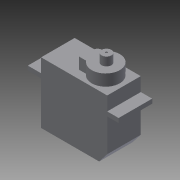
# Autodesk Inventor part: Part1
Saved by Autodesk Inventor 2015 (Build 190159000, 159)
## iProperties
Created: 2015-05-19
Part Number: Part1
Material: Generic
Document SubType Name: Modeling
Designer: Angelina
Density: 1 g/cm^3
Appearance: Default
Author: Angelina
Autodesk Inventor part; units mm, degrees
ref_plane "YZ Plane" through (0, 0, 0) normal (1, 0, 0) x (0, 1, 0)
ref_plane "XZ Plane" through (0, 0, 0) normal (0, 1, 0) x (-1, 0, 0)
ref_plane "XY Plane" through (0, 0, 0) normal (0, 0, 1) x (1, 0, 0)
sketch "Sketch1" plane through (0, 0, 0) normal (0, 0, 1) x (1, 0, 0)
  line L0 (0, 0) -> (23.114, 0)
  line L1 (23.114, 0) -> (23.114, 15.0368)
  line L2 (23.114, 15.0368) -> (0, 15.0368)
  line L3 (0, 15.0368) -> (0, 0)
  dimension "d0" = 15.0368
  dimension "d1" = 23.114
  constraints: 8 end point, 2 parallel, 1 horizontal, 1 perpendicular
  measures "d0" distance of L2.end L0.start
  measures "d1" distance of L0.start L0.end
extrude "Extrusion1" add sketch "Sketch1" along normal blind 11.7348
sketch "Sketch2" plane through (0, 0, 11.7348) normal (0, 0, 1) x (1, 0, 0)
  line L0 (23.114, 0) -> (23.114, 3.6138)
  line L1 (23.114, 0) -> (23.114, 15.0368) projected
  line L2 (0, 0) -> (23.114, 0) projected
  line L3 (20.3034, 0) -> (23.114, 0)
  line L4 (23.114, 3.6138) -> (20.3034, 0)
  constraints: 6 end point, 2 point on line, 1 collinear
extrude "Extrusion2" cut sketch "Sketch2" against normal blind 11.7348
sketch "Sketch3" plane through (0, 0, 11.7348) normal (0, 0, 1) x (1, 0, 0)
  line L0 (-4.6433, 16.5606) -> (27.1067, 16.5606)
  line L1 (27.1067, 16.5606) -> (27.1067, 15.0366)
  line L2 (27.1067, 15.0366) -> (-4.6433, 15.0366)
  line L3 (-4.6433, 15.0366) -> (-4.6433, 16.5606)
  line L4 (23.114, 15.0368) -> (0, 15.0368) projected
  point P0 (0, 0)
  dimension "d6" = 31.75
  dimension "d7" = 1.524
  constraints: 8 end point, 1 horizontal, 1 parallel, 1 perpendicular
  measures "d6" distance of L0.start L0.end
  measures "d7" distance of L0.end L1.end
extrude "Extrusion3" add sketch "Sketch3" against normal blind 11.7348
sketch "Sketch4" plane through (0, 0, 11.7348) normal (0, 0, 1) x (1, 0, 0)
  line L0 (-4.6433, 16.5606) -> (27.1067, 16.5606) projected
  line L1 (0, 16.5606) -> (23.1157, 16.5606)
  line L2 (23.1157, 16.5606) -> (23.1157, 21.3866)
  line L3 (23.1157, 21.3866) -> (0, 21.3866)
  line L4 (0, 21.3866) -> (0, 16.5606)
  point P0 (0, 0)
  dimension "d10" = 4.826
  constraints: 8 end point, 2 parallel, 1 horizontal, 1 perpendicular, 1 point on line
  measures "d10" distance of L1.end L2.end
extrude "Extrusion4" add sketch "Sketch4" against normal up to surface (11.7348 mm away)
sketch "Sketch5" plane through (0, 21.3866, 11.7348) normal (0, 1, 0) x (1, 0, 0)
  circle A0 centre (16.7403, 5.8674) radius 4.8959
  point P0 (0, 11.7348)
  dimension "d14" = 9.7917
  constraints: 1 centre point
  measures "d14" diameter of A0
extrude "Extrusion5" add sketch "Sketch5" along normal blind 3.9878
sketch "Sketch6" plane through (16.7403, 25.3744, 5.8674) normal (0, 1, 0) x (1, 0, 0)
  circle A0 centre (0, 0) radius 4.8958 projected
  arc A1 (-3.876, 2.991) -> (-5.6698, 0.5745) centre (-4.3859, 1.4955) ccw
  line L0 (-5.6698, 0.5745) -> (-6.3204, 0.5745)
  line L1 (-6.3204, 0.5745) -> (-6.3204, -2.991)
  line L2 (-6.3204, -2.991) -> (-3.876, -2.991)
  line L3 (-3.876, 0) -> (-3.876, 0.5745)
  point P0 (-16.7403, 5.8674)
  constraints: 8 end point, 5 point on circle, 2 parallel, 1 centre point, 1 horizontal, 1 perpendicular
extrude "Extrusion6" add sketch "Sketch6" against normal blind 3.9878 contours A0 L2 L1 L0 A1
sketch "Sketch7" plane through (0, 25.3744, 11.7348) normal (0, 1, 0) x (1, 0, 0)
  circle A0 centre (16.9713, 5.8977) radius 1.7145
  point P0 (0, 11.7348)
  dimension "d19" = 3.429
  constraints: 1 centre point, 1 coincident
  measures "d19" diameter of A0
extrude "Extrusion7" add sketch "Sketch7" along normal blind 2.9718
sketch "Sketch8" plane through (16.9713, 28.3462, 5.8371) normal (0, 1, 0) x (1, 0, 0)
  circle A0 centre (0, 0) radius 0.41
  point P0 (-16.9713, 5.8371)
  constraints: 1 centre point
extrude "Extrusion8" cut sketch "Sketch8" against normal blind 0.254
body "Solid1"
